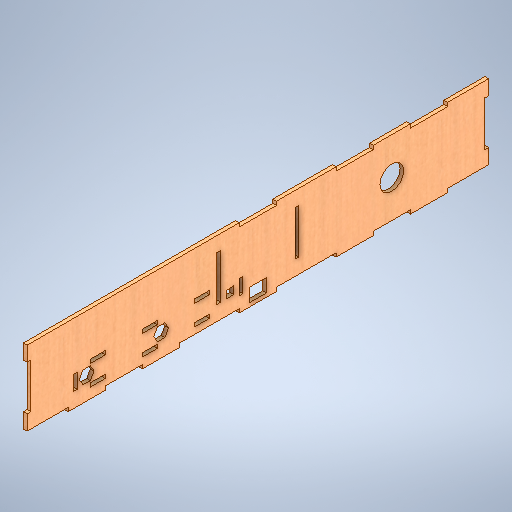
# Autodesk Inventor part: Lat2
Saved by Autodesk Inventor 2025 (Build 290162000, 162)
## iProperties
Created: 2024-11-02
Part Number: Lat2
Material: Wood (Cherry)
Document SubType Name: Sheet Metal
Designer: g.marin
Density: 0.63 g/cm^3
Sheet Metal Rule: Default
Appearance: Cherry - Natural Low Gloss
Author: g.marin
Autodesk Inventor part; units mm, degrees
ref_plane "YZ Plane" through (0, 0, 0) normal (1, 0, 0) x (0, 1, 0)
ref_plane "XZ Plane" through (0, 0, 0) normal (0, 1, 0) x (-1, 0, 0)
ref_plane "XY Plane" through (0, 0, 0) normal (0, 0, 1) x (1, 0, 0)
sketch "Sketch1" plane through (0, 0, 0) normal (1, 0, 0) x (0, 1, 0)
  line L0 (-50, 50) -> (50, 50)
  line L1 (50, 50) -> (50, -50)
  line L2 (50, -50) -> (-50, -50)
  line L3 (-50, -50) -> (-50, 50)
  line L4 (-50, 50) -> (50, -50) construction
  line L5 (50, 50) -> (-50, -50) construction
  line L6 (50, 50) -> (-50, 50)
  line L7 (-50, 50) -> (-50, 310)
  line L8 (-50, 310) -> (50, 310)
  line L9 (50, 310) -> (50, 50)
  line L10 (50, -50) -> (-50, -50)
  line L11 (-50, -50) -> (-50, -310)
  line L12 (-50, -310) -> (50, -310)
  line L13 (50, -310) -> (50, -50)
  line L14 (-50, 255) -> (-55, 255)
  line L15 (-55, 255) -> (-55, 205)
  line L16 (-55, 205) -> (-50, 205)
  line L17 (-50, 205) -> (-50, 255)
  line L18 (-50, 155) -> (-55, 155)
  line L19 (-55, 155) -> (-55, 105)
  line L20 (-55, 105) -> (-50, 105)
  line L21 (-50, 105) -> (-50, 155)
  line L22 (-50, 25) -> (-55, 25)
  line L23 (-55, 25) -> (-55, -25)
  line L24 (-55, -25) -> (-50, -25)
  line L25 (-50, -25) -> (-50, 25)
  line L26 (-50, -105) -> (-55, -105)
  line L27 (-55, -105) -> (-55, -155)
  line L28 (-55, -155) -> (-50, -155)
  line L29 (-50, -155) -> (-50, -105)
  line L30 (-50, -205) -> (-55, -205)
  line L31 (-55, -205) -> (-55, -255)
  line L32 (-55, -255) -> (-50, -255)
  line L33 (-50, -255) -> (-50, -205)
  line L34 (50, 310) -> (30, 310)
  line L35 (50, 305) -> (50, 310)
  line L36 (-50, 310) -> (-30, 310)
  line L37 (-50, 305) -> (-50, 310)
  line L38 (30, 50) -> (-30, 50)
  line L39 (-30, 50) -> (-30, 55)
  line L40 (-30, 55) -> (30, 55)
  line L41 (30, 55) -> (30, 50)
  line L42 (30, -50) -> (-36.1124, -50)
  line L43 (50, 0) -> (-50, 0) construction
  line L44 (-30, -50) -> (-30, -55)
  line L45 (-30, -55) -> (30, -55)
  line L46 (30, -55) -> (30, -50)
  line L47 (30, 310) -> (-30, 310)
  line L48 (-30, 310) -> (-30, 305)
  line L49 (-30, 305) -> (30, 305)
  line L50 (30, 305) -> (30, 310)
  line L51 (-30, -310) -> (-30, -305)
  line L52 (-30, -305) -> (30, -305)
  line L53 (30, -305) -> (30, -310)
  line L54 (-50, -180) -> (50, -180) construction
  circle A0 centre (0, -180) radius 16
  line L55 (50, 25) -> (45, 25)
  line L56 (45, 25) -> (45, -25)
  line L57 (45, -25) -> (50, -25)
  line L58 (50, -25) -> (50, 25)
  line L59 (50, -105) -> (45, -105)
  line L60 (45, -105) -> (45, -155)
  line L61 (45, -155) -> (50, -155)
  line L62 (50, -155) -> (50, -105)
  line L63 (50, -255) -> (45, -255)
  line L64 (45, -255) -> (45, -205)
  line L65 (45, -205) -> (50, -205)
  line L66 (-50, 11.5) -> (-32, 11.5)
  line L67 (-32, 11.5) -> (-32, -11.5)
  line L68 (-32, -11.5) -> (-50, -11.5)
  line L69 (-50, -11.5) -> (-50, 11.5)
  line L70 (-33.6603, 235) -> (-25, 240)
  line L71 (-25, 240) -> (-16.3397, 235)
  line L72 (-16.3397, 235) -> (-16.3397, 225)
  line L73 (-16.3397, 225) -> (-25, 220)
  line L74 (-25, 220) -> (-33.6603, 225)
  line L75 (-33.6603, 225) -> (-33.6603, 235)
  line L76 (-33.6603, 135) -> (-25, 140)
  line L77 (-25, 140) -> (-16.3397, 135)
  line L78 (-16.3397, 135) -> (-16.3397, 125)
  line L79 (-16.3397, 125) -> (-25, 120)
  line L80 (-25, 120) -> (-33.6603, 125)
  line L81 (-33.6603, 125) -> (-33.6603, 135)
  line L82 (-8.75, 225) -> (-13.75, 225)
  line L83 (-13.75, 225) -> (-13.75, 205)
  line L84 (-13.75, 205) -> (-8.75, 205)
  line L85 (-8.75, 205) -> (-8.75, 225)
  line L86 (-13.75, 135) -> (-8.75, 135)
  line L87 (-8.75, 135) -> (-8.75, 155)
  line L88 (-8.75, 155) -> (-13.75, 155)
  line L89 (-13.75, 155) -> (-13.75, 135)
  line L90 (-13.75, 85) -> (-8.75, 85)
  line L91 (-8.75, 85) -> (-8.75, 65)
  line L92 (-8.75, 65) -> (-13.75, 65)
  line L93 (-13.75, 65) -> (-13.75, 85)
  line L94 (-25, 314.14) -> (-25, -94.5604) construction
  line L95 (-41.25, 225) -> (-36.25, 225)
  line L96 (-36.25, 225) -> (-36.25, 205)
  line L97 (-36.25, 205) -> (-41.25, 205)
  line L98 (-41.25, 205) -> (-41.25, 225)
  line L99 (-36.25, 135) -> (-41.25, 135)
  line L100 (-41.25, 135) -> (-41.25, 155)
  line L101 (-41.25, 155) -> (-36.25, 155)
  line L102 (-36.25, 155) -> (-36.25, 135)
  line L103 (-36.25, 85) -> (-41.25, 85)
  line L104 (-41.25, 85) -> (-41.25, 65)
  line L105 (-41.25, 65) -> (-36.25, 65)
  line L106 (-36.25, 65) -> (-36.25, 85)
  line L107 (-15, 242.5) -> (-35, 242.5)
  line L108 (-35, 242.5) -> (-35, 247.5)
  line L109 (-35, 247.5) -> (-15, 247.5)
  line L110 (-15, 247.5) -> (-15, 242.5)
  line L111 (-15, 20) -> (-35, 20)
  line L112 (-35, 20) -> (-35, 25)
  line L113 (-35, 25) -> (-15, 25)
  line L114 (-15, 25) -> (-15, 20)
  line L115 (-20, 42.5) -> (-30, 42.5)
  line L116 (-30, 42.5) -> (-30, 32.5)
  line L117 (-30, 32.5) -> (-20, 32.5)
  line L118 (-20, 32.5) -> (-20, 42.5)
  point P0 (0, 0)
  point P1 (-52.5, 155)
  point P2 (-52.5, 205)
  point P3 (-50, 205)
  point P4 (-50, 105)
  point P5 (-50, -155)
  point P6 (-50, -255)
  point P7 (30, -50)
  point P8 (-30, -50)
  point P9 (-30, 50)
  point P10 (30, 50)
  point P11 (30, 307.5)
  point P12 (-30, -310)
  point P13 (30, -310)
  point P14 (30, 310)
  point P15 (-30, 310)
  point P16 (50, -25)
  point P17 (50, -255)
  point P18 (50, -205)
  point P19 (50, -155)
  point P20 (-50, 0)
  point P21 (-50, 11.5)
  point P22 (-50, -11.5)
  point P23 (-25, 230)
  point P24 (-25, 130)
  point P25 (-13.75, 145)
  point P26 (-36.25, 145)
  point P27 (-15, 22.5)
  point P28 (-30, 37.5)
  dimension "d0" = 100
  dimension "d1" = 260
  dimension "d2" = 100
  dimension "d3" = 260
  dimension "d4" = 50
  dimension "d5" = 50
  dimension "d6" = 50
  dimension "d7" = 50
  dimension "d8" = 50
  dimension "d9" = 55
  dimension "d10" = 50
  dimension "d11" = 25
  dimension "d12" = 55
  dimension "d13" = 50
  dimension "d14" = 5
  dimension "d20" = 5
  dimension "d21" = 5
  dimension "d23" = 20
  dimension "d26" = 32
  dimension "d27" = 5
  dimension "d28" = 5
  dimension "d29" = 18
  dimension "d30" = 23
  dimension "d31" = 11.5
  dimension "d32" = 20
  dimension "d34" = 10
  dimension "d35" = 25
  dimension "d37" = 25
  dimension "d38" = 16.3397
  dimension "d39" = 10
  dimension "d40" = 25
  dimension "d41" = 16.3397
  dimension "d42" = 25
  dimension "d43" = 11.25
  dimension "d44" = 20
  dimension "d45" = 0
  dimension "d46" = 5
  dimension "d47" = 20
  dimension "d48" = 5
  dimension "d49" = 11.25
  dimension "d50" = 50
  dimension "d51" = 20
  dimension "d52" = 5
  dimension "d53" = 11.25
  dimension "d54" = 11.25
  dimension "d55" = 20
  dimension "d56" = 10
  dimension "d57" = 5
  dimension "d58" = 12.5
  dimension "d59" = 5
  dimension "d60" = 20
  dimension "d61" = 10
  dimension "d62" = 40
  dimension "d63" = 10
  dimension "d64" = 10
  dimension "d65" = 5
  dimension "d66" = 7.5
  constraints: 238 end point, 38 parallel, 24 symmetric about line, 22 horizontal, 19 perpendicular, 16 point on line, 14 midpoint, 8 collinear, 1 centre point, 1 vertical, 26 other
  measures "d0" distance of L11.end L12.end
  measures "d1" distance of L12.end L1.end
  measures "d2" distance of L0.end L1.end
  measures "d3" distance of L8.end L0.end
  measures "d4" distance of L14.end L15.end
  measures "d5" distance of L18.end L19.end
  measures "d6" distance of L22.end L23.end
  measures "d7" distance of L26.end L27.end
  measures "d8" distance of L30.end L31.end
  measures "d9" vertical distance of L14.end L7.end
  measures "d10" distance of point (-52.5, 155) point (-52.5, 205)
  measures "d11" vertical distance of L22.end L0.start
  measures "d12" vertical distance of L26.end L2.end
  measures "d13" distance of L30.end L27.end
  measures "d14" distance of L14.start L14.end
  measures "d20" distance between parallel lines of L0 L40
  measures "d21" distance of L49.end L34.end
  measures "d23" distance from line of point (30, 307.5) L9
  measures "d26" diameter of A0
  measures "d27" distance between parallel lines of L56 L58
  measures "d28" distance between parallel lines of L62 L60
  measures "d29" distance of L67.end L68.end
  measures "d30" distance of L66.end L67.end
  measures "d31" distance from line of point (-50, 0) L66
  measures "d32" distance between parallel lines of L37 L48
  measures "d34" distance of L74.end L70.start
  measures "d35" distance from line of L17 point (-25, 230)
  measures "d37" distance from line of point (-25, 230) L14
  measures "d38" distance from line of L17 L70.start
  measures "d39" distance of L81.start L76.start
  measures "d40" distance from line of L7 point (-25, 130)
  measures "d41" distance from line of L21 L81.start
  measures "d42" horizontal distance of L18.start point (-25, 130)
  measures "d43" distance from line of L83 point (-25, 230)
  measures "d44" distance between parallel lines of L84 L82
  measures "d45" distance from line of L72.end L82
  measures "d46" distance between parallel lines of L85 L83
  measures "d47" distance of L86.end L87.end
  measures "d48" distance of L86.start L86.end
  measures "d49" horizontal distance of point (-25, 130) point (-13.75, 145)
  measures "d50" distance of L90.end L86.end
  measures "d51" distance of L90.end L91.end
  measures "d52" distance of L91.end L92.end
  measures "d53" distance from line of point (-25, 130) L93
  measures "d54" distance between parallel lines of L94 L96
  measures "d55" distance of L108.end L109.end
  measures "d56" distance between parallel lines of L94 L110
  measures "d57" distance of L109.end L107.start
  measures "d58" distance from line of L107 point (-25, 230)
  measures "d59" distance between parallel lines of L113 L111
  measures "d60" distance of L111.start L111.end
  measures "d61" distance from line of L94 point (-15, 22.5)
  measures "d62" vertical distance of L112.end L106.start
  measures "d63" distance of L117.end L115.start
  measures "d64" distance of L116.end L117.end
  measures "d65" distance from line of L94 point (-30, 37.5)
  measures "d66" distance of L115.end L38.end
extrude "Extrusion1" add sketch "Sketch1" along normal blind 5 contours L7 L8 L48 L49 L50 L9 L0 L41 L40 L39 | L0 L1 L55 L56 L57 L2 L3 L68 L67 L66 | L3 L24 L23 L22 | L20 L19 L18 L7 | L16 L15 L14 L7 | L2 L44 L45 L46 L13 L59 L60 L61 L65 L64 L63 L12 L53 L52 L51 L11 | L11 L28 L27 L26 | L11 L32 L31 L30
equation "\"BendRadius\" = Thickness"
equation "\"BendReliefWidth\" = Thickness"
equation "\"BendReliefDepth\" = 0.5 * Thickness"
equation "\"CornerReliefSize\" = 4 * Thickness"
equation "\"MinimumRemnant\" = 2 * Thickness"
equation "\"TransitionRadius\" = BendRadius"
equation "\"JacobiRadiusSize\" = BendRadius"
equation "\"GapSize\" = Thickness"
equation "\"Thickness\" = 3.048"
body "Solid1" dims "d8" = 50
